Autodesk Inventor part; units mm, degrees
(part 2 of 2)
  line L321 (44.905, -4.4402) -> (43.7756, -7.9673)
  line L322 (43.7756, -7.9673) -> (42.4567, -7.9673)
  line L323 (39.3847, -2.7673) -> (42.1828, -2.7673)
  line L324 (42.1828, -2.7673) -> (42.1828, -3.6733)
  line L325 (42.1828, -3.6733) -> (41.4369, -3.6733)
  line L326 (41.4369, -3.6733) -> (41.4369, -7.0613)
  line L327 (41.4369, -7.0613) -> (42.1828, -7.0613)
  line L328 (42.1828, -7.0613) -> (42.1828, -7.9673)
  line L329 (42.1828, -7.9673) -> (39.3847, -7.9673)
  line L330 (39.3847, -7.9673) -> (39.3847, -7.0613)
  line L331 (39.3847, -7.0613) -> (40.1306, -7.0613)
  line L332 (40.1306, -7.0613) -> (40.1306, -3.6733)
  line L333 (40.1306, -3.6733) -> (39.3847, -3.6733)
  line L334 (39.3847, -3.6733) -> (39.3847, -2.7673)
  line L335 (37.5179, -2.7673) -> (37.5179, -6.977)
  line L336 (37.5179, -6.977) -> (39.056, -6.977)
  line L337 (39.056, -6.977) -> (39.056, -7.9673)
  line L338 (39.056, -7.9673) -> (34.6735, -7.9673)
  line L339 (34.6735, -7.9673) -> (34.6735, -6.977)
  line L340 (34.6735, -6.977) -> (36.2116, -6.977)
  line L341 (36.2116, -6.977) -> (36.2116, -2.7673)
  line L342 (36.2116, -2.7673) -> (37.5179, -2.7673)
  line L343 (28.2346, -2.7673) -> (32.0567, -2.7673)
  line L344 (32.0567, -2.7673) -> (32.0567, -3.6143)
  spline S200 degree 2 poles (32.0567, -3.6143) (31.5721, -4.002) (30.7967, -4.6847) (30.506, -4.9923) knots 0 0 0 1 2 2 2
  spline S201 degree 2 poles (30.506, -4.9923) (30.1225, -5.3926) (29.7812, -6.0036) (29.7812, -6.3239) knots 0 0 0 1 2 2 2
  spline S202 degree 2 poles (29.7812, -6.3239) (29.7812, -6.6863) (30.2152, -7.074) (30.6029, -7.074) knots 0 0 0 1 2 2 2
  spline S203 degree 2 poles (30.6029, -7.074) (30.8009, -7.074) (31.1549, -6.977) (31.3361, -6.9012) knots 0 0 0 1 2 2 2
  spline S204 degree 2 poles (31.3361, -6.9012) (31.5131, -6.8211) (31.7659, -6.6526) (31.8291, -6.6104) knots 0 0 0 1 2 2 2
  line L345 (31.8291, -6.6104) -> (31.9303, -6.6104)
  line L346 (31.9303, -6.6104) -> (31.9303, -7.744)
  spline S205 degree 2 poles (31.9303, -7.744) (31.7111, -7.8493) (30.7756, -8.0684) (30.3416, -8.0684) knots 0 0 0 1 2 2 2
  spline S206 degree 2 poles (30.3416, -8.0684) (29.4145, -8.0684) (28.4622, -7.2425) (28.4622, -6.4966) knots 0 0 0 1 2 2 2
  spline S207 degree 2 poles (28.4622, -6.4966) (28.4622, -6.0373) (28.8962, -5.1524) (29.3977, -4.6467) knots 0 0 0 1 2 2 2
  spline S208 degree 2 poles (29.3977, -4.6467) (29.7137, -4.3349) (30.3079, -3.8503) (30.4385, -3.7492) knots 0 0 0 1 2 2 2
  line L347 (30.4385, -3.7492) -> (28.2346, -3.7492)
  line L348 (28.2346, -3.7492) -> (28.2346, -2.7673)
  spline S209 degree 2 poles (23.7468, -5.3673) (23.7468, -4.6931) (23.9617, -3.6817) (24.2019, -3.3404) knots 0 0 0 1 2 2 2
  spline S210 degree 2 poles (24.2019, -3.3404) (24.4379, -3.0033) (25.2006, -2.6578) (25.7484, -2.6578) knots 0 0 0 1 2 2 2
  spline S211 degree 2 poles (25.7484, -2.6578) (26.3004, -2.6578) (27.0589, -3.0033) (27.2991, -3.3488) knots 0 0 0 1 2 2 2
  spline S212 degree 2 poles (27.2991, -3.3488) (27.5393, -3.6902) (27.7542, -4.6931) (27.7542, -5.3673) knots 0 0 0 1 2 2 2
  spline S213 degree 2 poles (27.7542, -5.3673) (27.7542, -6.0584) (27.5393, -7.036) (27.2949, -7.39) knots 0 0 0 1 2 2 2
  spline S214 degree 2 poles (27.2949, -7.39) (27.0505, -7.7355) (26.2794, -8.0727) (25.7484, -8.0727) knots 0 0 0 1 2 2 2
  spline S215 degree 2 poles (25.7484, -8.0727) (25.188, -8.0727) (24.4379, -7.7187) (24.1977, -7.3689) knots 0 0 0 1 2 2 2
  spline S216 degree 2 poles (24.1977, -7.3689) (23.9617, -7.0276) (23.7468, -6.0205) (23.7468, -5.3673) knots 0 0 0 1 2 2 2
  spline S217 degree 2 poles (25.0573, -5.3673) (25.0573, -6.3323) (25.3734, -7.1119) (25.7484, -7.1119) knots 0 0 0 1 2 2 2
  spline S218 degree 2 poles (25.7484, -7.1119) (26.1235, -7.1119) (26.4437, -6.3323) (26.4437, -5.3631) knots 0 0 0 1 2 2 2
  spline S219 degree 2 poles (26.4437, -5.3631) (26.4437, -4.4107) (26.1235, -3.6185) (25.7484, -3.6185) knots 0 0 0 1 2 2 2
  spline S220 degree 2 poles (25.7484, -3.6185) (25.3776, -3.6185) (25.0573, -4.4107) (25.0573, -5.3673) knots 0 0 0 1 2 2 2
  line L349 (19.3559, -2.7673) -> (22.7902, -2.7673)
  line L350 (22.7902, -2.7673) -> (22.7902, -3.6733)
  line L351 (22.7902, -3.6733) -> (21.6946, -3.6733)
  line L352 (21.6946, -3.6733) -> (21.6946, -6.425)
  line L353 (21.6946, -6.425) -> (22.7902, -6.425)
  line L354 (22.7902, -6.425) -> (22.7902, -7.272)
  spline S221 degree 2 poles (22.7902, -7.272) (22.55, -7.272) (22.0739, -7.3352) (21.9306, -7.4026) knots 0 0 0 1 2 2 2
  spline S222 degree 2 poles (21.9306, -7.4026) (21.7662, -7.4869) (21.5808, -7.7693) (21.564, -7.98) knots 0 0 0 1 2 2 2
  line L355 (21.564, -7.98) -> (20.4262, -7.98)
  line L356 (20.4262, -7.98) -> (20.4262, -3.6733)
  line L357 (20.4262, -3.6733) -> (19.3559, -3.6733)
  line L358 (19.3559, -3.6733) -> (19.3559, -2.7673)
  spline S223 degree 2 poles (14.7037, -5.6581) (14.7037, -4.9965) (15.0113, -3.8924) (15.3358, -3.4963) knots 0 0 0 1 2 2 2
  spline S224 degree 2 poles (15.3358, -3.4963) (15.6729, -3.096) (16.6674, -2.6662) (17.3922, -2.6662) knots 0 0 0 1 2 2 2
  spline S225 degree 2 poles (17.3922, -2.6662) (17.6366, -2.6662) (18.1675, -2.7294) (18.256, -2.7547) knots 0 0 0 1 2 2 2
  line L359 (18.256, -2.7547) -> (18.256, -3.7744)
  line L360 (18.256, -3.7744) -> (18.1549, -3.7744)
  spline S226 degree 2 poles (18.1549, -3.7744) (18.058, -3.7239) (17.6956, -3.6143) (17.3795, -3.6143) knots 0 0 0 1 2 2 2
  spline S227 degree 2 poles (17.3795, -3.6143) (17.1225, -3.6143) (16.6463, -3.7492) (16.4778, -3.8966) knots 0 0 0 1 2 2 2
  spline S228 degree 2 poles (16.4778, -3.8966) (16.2966, -4.0526) (16.0606, -4.5119) (16.0184, -4.8574) knots 0 0 0 1 2 2 2
  spline S229 degree 2 poles (16.0184, -4.8574) (16.2966, -4.6847) (16.7769, -4.4992) (17.1351, -4.4992) knots 0 0 0 1 2 2 2
  spline S230 degree 2 poles (17.1351, -4.4992) (17.4006, -4.4992) (17.8936, -4.6425) (18.0959, -4.7942) knots 0 0 0 1 2 2 2
  spline S231 degree 2 poles (18.0959, -4.7942) (18.3656, -5.0007) (18.6816, -5.6623) (18.6816, -6.1848) knots 0 0 0 1 2 2 2
  spline S232 degree 2 poles (18.6816, -6.1848) (18.6816, -6.5936) (18.4035, -7.2804) (18.1507, -7.5333) knots 0 0 0 1 2 2 2
  spline S233 degree 2 poles (18.1507, -7.5333) (17.8978, -7.7861) (17.1646, -8.0727) (16.7137, -8.0727) knots 0 0 0 1 2 2 2
  spline S234 degree 2 poles (16.7137, -8.0727) (16.2586, -8.0727) (15.5549, -7.8198) (15.3021, -7.5543) knots 0 0 0 1 2 2 2
  spline S235 degree 2 poles (15.3021, -7.5543) (15.0071, -7.2594) (14.7037, -6.3239) (14.7037, -5.6581) knots 0 0 0 1 2 2 2
  spline S236 degree 2 poles (15.9974, -5.8519) (15.9974, -6.2775) (16.1406, -6.8253) (16.2713, -6.977) knots 0 0 0 1 2 2 2
  spline S237 degree 2 poles (16.2713, -6.977) (16.3598, -7.0908) (16.5873, -7.1877) (16.7179, -7.1877) knots 0 0 0 1 2 2 2
  spline S238 degree 2 poles (16.7179, -7.1877) (16.8359, -7.1877) (17.0551, -7.095) (17.1562, -6.977) knots 0 0 0 1 2 2 2
  spline S239 degree 2 poles (17.1562, -6.977) (17.2447, -6.8759) (17.3711, -6.484) (17.3711, -6.2522) knots 0 0 0 1 2 2 2
  spline S240 degree 2 poles (17.3711, -6.2522) (17.3711, -5.9994) (17.2405, -5.6749) (17.1309, -5.578) knots 0 0 0 1 2 2 2
  spline S241 degree 2 poles (17.1309, -5.578) (17.0171, -5.4811) (16.7348, -5.4052) (16.5578, -5.4052) knots 0 0 0 1 2 2 2
  spline S242 degree 2 poles (16.5578, -5.4052) (16.4103, -5.4052) (16.1027, -5.4853) (16.0058, -5.5274) knots 0 0 0 1 2 2 2
  spline S243 degree 2 poles (16.0058, -5.5274) (16.0058, -5.5654) (15.9974, -5.7086) (15.9974, -5.8519) knots 0 0 0 1 2 2 2
  constraints: 2 other
extrude "Extrusion3" cut sketch "Sketch3" against normal blind 10
body "Solid1"
